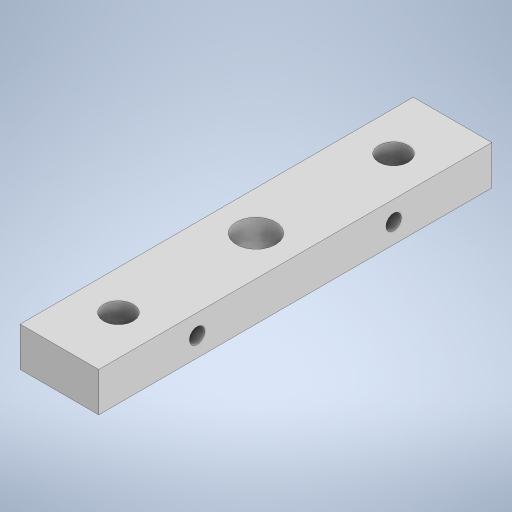
# Autodesk Inventor part: Metal Bar-2
Saved by Autodesk Inventor 2024 (Build 280153000, 153)
## iProperties
Created: 2024-03-20
Part Number: Metal Bar-2
Material: Generic
Document SubType Name: Modeling
Designer: Liz
Density: 1 g/cm^3
Appearance: Default
Author: Liz
Autodesk Inventor part; units mm, degrees
ref_plane "YZ Plane" through (0, 0, 0) normal (1, 0, 0) x (0, 1, 0)
ref_plane "XZ Plane" through (0, 0, 0) normal (0, 1, 0) x (-1, 0, 0)
ref_plane "XY Plane" through (0, 0, 0) normal (0, 0, 1) x (1, 0, 0)
sketch "Sketch1" plane through (0, 0, 0) normal (0, 0, 1) x (1, 0, 0)
  line L0 (-25.4, -12.7) -> (25.4, -12.7)
  line L1 (25.4, -12.7) -> (25.4, 12.7)
  line L2 (25.4, 12.7) -> (-25.4, 12.7)
  line L3 (-25.4, 12.7) -> (-25.4, -12.7)
  line L4 (-25.4, -12.7) -> (25.4, 12.7) construction
  line L5 (25.4, -12.7) -> (-25.4, 12.7) construction
  point P0 (0, 0)
  dimension "d0" = 25.4
  dimension "d1" = 50.8
  constraints: 12 end point, 2 midpoint, 2 parallel, 1 horizontal, 1 perpendicular
  measures "d0" distance of L2.end L0.start
  measures "d1" distance of L1.end L2.end
extrude "Extrusion1" add sketch "Sketch1" against normal blind 254
sketch "Sketch2" plane through (-25.4, 12.7, 0) normal (0, 1, 0) x (1, 0, 0)
  circle A0 centre (25.4, 38.1) radius 9.525
  circle A1 centre (25.4, 215.9) radius 9.525
  line L0 (50.8, 0) -> (0, 0) projected
  line L1 (0, 0) -> (0, 254) projected
  circle A2 centre (25.4, 127) radius 12.7
  point P0 (25.4, 0)
  point P1 (25.4, 0)
  point P2 (0, 127)
  point P3 (0, 127)
  dimension "d4" = 19.05
  dimension "d5" = 88.9
  dimension "d6" = 177.8
  dimension "d9" = 25.4
  constraints: 3 centre point, 3 midpoint, 3 vertical alignment, 1 equal radius, 1 horizontal alignment
  measures "d4" diameter of A0
  measures "d5" vertical distance of point (0, 127) A0.centre
  measures "d6" distance of A0.centre A1.centre
  measures "d9" diameter of A2
extrude "Extrusion2" cut sketch "Sketch2" against normal blind 254
sketch "Sketch3" plane through (25.4, -12.7, 0) normal (1, 0, 0) x (0, 0, -1)
  circle A0 centre (63.5, 12.7) radius 5
  circle A1 centre (190.5, 12.7) radius 5
  line L0 (0, 25.4) -> (254, 25.4) projected
  line L1 (0, 0) -> (0, 25.4) projected
  point P0 (0, 12.7)
  point P1 (127, 25.4)
  point P2 (0, 12.7)
  dimension "d10" = 10
  dimension "d11" = 127
  dimension "d12" = 63.5
  constraints: 2 centre point, 2 horizontal alignment, 2 midpoint, 1 equal radius
  measures "d10" diameter of A0
  measures "d11" distance of A1.centre A0.centre
  measures "d12" horizontal distance of point (127, 25.4) A0.centre
extrude "Extrusion3" cut sketch "Sketch3" against normal blind 254
body "Solid1"
